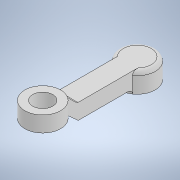
# Autodesk Inventor part: Рулевая тяга левая
Saved by Autodesk Inventor 2020 (Build 240168000, 168)
## iProperties
Created: 2021-08-11
Part Number: Рулевая тяга левая
Material: Типовые
Document SubType Name: Обычные детали
Designer: Антон
Density: 1 g/cm^3
Appearance: По умолчанию
Sheet Metal Rule: По умолчанию
Author: Антон
Autodesk Inventor part; units mm, degrees
ref_plane "YZ Plane" through (0, 0, 0) normal (1, 0, 0) x (0, 1, 0)
ref_plane "XZ Plane" through (0, 0, 0) normal (0, 1, 0) x (-1, 0, 0)
sketch "Эскиз6" plane through (0, 0, 0) normal (0, 1, 0) x (-1, 0, 0)
  circle A0 centre (0, 0) radius 2.575
  circle A1 centre (0, 0) radius 4.575
  dimension "d11" = 5.15
  dimension "d12" = 2
  constraints: 2 centre point, 2 coincident
  measures "d11" diameter of A0
  measures "d12" radial gap between concentric circles of A1 A0
extrude "Выдавливание5" add sketch "Эскиз6" along normal blind 4
ref_plane "РабПлоскость1" through (0, 1.6, 0) normal (0, -1, 0) x (1, 0, 0)
sketch "Эскиз1" plane through (0, 1.6, 0) normal (0, 1, 0) x (-1, 0, 0)
  circle A0 centre (0, 0) radius 2.575 projected
  line L0 (-2.575, 0) -> (2.575, 0)
  line L1 (2.575, 0) -> (2.575, -24.1495)
  line L2 (2.575, -24.1495) -> (-2.575, -24.1495)
  line L3 (-2.575, -24.1495) -> (-2.575, 0)
  circle A1 centre (0, -24.1495) radius 4.575
  circle A2 centre (0, 0) radius 4.575 projected
  circle A3 centre (0, 0) radius 4.575 projected
  circle A4 centre (0, 0) radius 4.575 projected
  circle A5 centre (0, 0) radius 2.575 projected
  point P0 (2.575, -3.7815)
  point P1 (-2.575, -3.7815)
  point P2 (-2.575, -20.3679)
  point P3 (2.575, -20.3679)
  dimension "d15" = 24.1495
  constraints: 8 end point, 2 midpoint, 2 parallel, 1 centre point, 1 coincident, 1 equal radius, 1 horizontal, 1 perpendicular, 1 tangent
  measures "d15" distance of L2.end L0.start
extrude "Выдавливание1" add sketch "Эскиз1" against normal blind 4 separate body contours L1 A1 L3 A2 | A1 L3 L2 L1 | L1 L2 L3 A1
sketch "Эскиз9" plane through (0, 1.6, 0) normal (0, 1, 0) x (1, 0, 0)
  circle A0 centre (0, 0) radius 4.575 projected
  circle A1 centre (0, 0) radius 2.575 projected
  circle A2 centre (0, 0) radius 2.575 projected
  line L0 (-2.575, 3.7815) -> (-2.575, 20.3679) projected
  line L1 (2.575, 0) -> (-2.575, 0)
  line L2 (-2.575, 0) -> (-2.575, 5.975)
  line L3 (-2.575, 5.975) -> (2.575, 5.975)
  line L4 (2.575, 5.975) -> (2.575, 0)
  line L5 (2.575, 3.7815) -> (2.575, 20.3679) projected
  dimension "d26" = 5.975
  constraints: 8 end point, 2 parallel, 1 collinear, 1 horizontal, 1 horizontal alignment, 1 perpendicular, 1 point on line, 1 other
  measures "d26" distance from line of L3 A0.centre
extrude "Выдавливание8" add sketch "Эскиз9" along normal up to surface (2.4 mm away) contours A0 L0 L3 L4 bodies 2
chamfer "Фаска2" distance 2.193 angle 45 1 edges at (0, 4, -5.975)
fillet "Сопряжение4" radius 0.621 1 edges at (0, 1.6, -5.975)
chamfer "Фаска1" distance 2.4 angle 45 1 edges at (0, -2.4, -4.575)
sketch "Эскиз7" plane through (0, -2.4, 0) normal (0, -1, 0) x (1, 0, 0)
  arc A0 (-2.575, -20.3679) -> (2.575, -20.3679) centre (0, -24.1495) ccw projected
  circle A1 centre (0, -24.1495) radius 4.575
  point P0 (0, 0)
  point P1 (-2.575, -20.3679)
  constraints: 1 coincident, 3 other
extrude "Выдавливание6" add sketch "Эскиз7" along normal blind 1.1 bodies 2
sketch "Эскиз8" plane through (0, -3.5, -24.1495) normal (0, -1, 0) x (1, 0, 0)
  circle A0 centre (0, 0) radius 4.575 projected
  circle A1 centre (0, 0) radius 2.575
  circle A2 centre (0, 24.1495) radius 2.575 projected
  constraints: 1 centre point, 1 coincident, 1 equal radius
extrude "Выдавливание7" cut sketch "Эскиз8" against normal blind 4 contours A1 bodies 2
fillet "Сопряжение1" radius 1.1 1 edges at (0, -2.4, -19.5745)
fillet "Сопряжение2" radius 1 1 edges at (0, 1.6, -28.7245)
equation "\"Радиус_гибки\" = Толщина"
equation "\"Ширина_просечки\" = Толщина"
equation "\"Глубина_просечки\" = 0.5 * Толщина"
equation "\"Размер_просечки\" = 4 * Толщина"
equation "\"Мин_остаток\" = 2 * Толщина"
equation "\"Радиус_перехода\" = Радиус_гибки"
equation "\"Радиус_Якоби\" = Толщина"
equation "\"Размер_зазора\" = Толщина"
equation "\"Толщина\" = 0.5"
